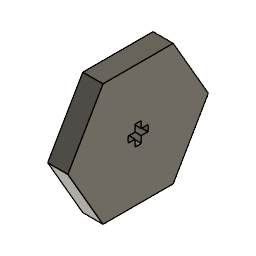
Hexagon cap (Autodesk Fusion 360 design; units mm, degrees)
part number: 2026-06-06-23-04-54-511
Autodesk Fusion 360 part; units mm, degrees
sketch "Sketch1" plane through (0, 0, 0) normal (1, 0, 0) x (0, 1, 0)
  line L0 (-1.7321, 3) -> (-3.4641, 0)
  line L1 (-3.4641, 0) -> (-1.7321, -3)
  line L2 (-1.7321, -3) -> (1.7321, -3)
  line L3 (1.7321, -3) -> (3.4641, 0)
  line L4 (3.4641, 0) -> (1.7321, 3)
  line L5 (1.7321, 3) -> (-1.7321, 3)
  line L6 (0.15, 0.15) -> (0.15, 0.477)
  line L7 (0.15, 0.15) -> (0.477, 0.15)
  line L8 (0.15, -0.15) -> (0.477, -0.15)
  line L9 (-0.15, 0.15) -> (-0.15, 0.477)
  line L10 (-0.15, 0.15) -> (-0.477, 0.15)
  line L11 (-0.15, -0.15) -> (-0.15, -0.477)
  line L12 (-0.15, -0.15) -> (-0.477, -0.15)
  line L13 (0.15, -0.15) -> (0.15, -0.477)
  arc A0 (0.477, -0.15) -> (0.477, 0.15) centre (0, 0) ccw
  arc A1 (-0.15, -0.477) -> (0.15, -0.477) centre (0, 0) ccw
  arc A2 (0.15, 0.477) -> (-0.15, 0.477) centre (0, 0) ccw
  arc A3 (-0.477, 0.15) -> (-0.477, -0.15) centre (0, 0) ccw
  dimension "d6" = 0.3
  constraint coincident A0.centre A1.centre
  constraint perpendicular L6 L7
  constraint concentric A0 A2
  constraint concentric A1 A3
  constraint concentric A2 A3
  measures "d6" distance of L6.start L8.start
extrude "Extrude1" add sketch "Sketch1" along normal blind 1
fillet "Fillet1" radius 0.1 12 edges at (0, -0.3135, -0.15) (0, -0.15, -0.3135) (0, 0, -0.5) (0, 0.15, -0.3135) (0, 0.3135, -0.15) (0, 0.5, 0) (0, 0.3135, 0.15) (0, 0.15, 0.3135) (0, 0, 0.5) (0, -0.15, 0.3135) (0, -0.3135, 0.15) (0, -0.5, 0)
